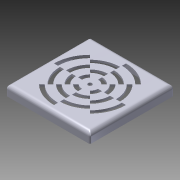
# Autodesk Inventor part: CompCellScopeArrayCover
Saved by Autodesk Inventor 2015 (Build 190159000, 159)
## iProperties
Created: 2015-03-24
Part Number: CompCellScopeArrayCover
Material: Generic
Document SubType Name: Modeling
Designer: Nitin
Density: 1 g/cm^3
Appearance: Default
Author: Nitin
Autodesk Inventor part; units mm, degrees
ref_plane "YZ Plane" through (0, 0, 0) normal (1, 0, 0) x (0, 1, 0)
ref_plane "XZ Plane" through (0, 0, 0) normal (0, 1, 0) x (-1, 0, 0)
ref_plane "XY Plane" through (0, 0, 0) normal (0, 0, 1) x (1, 0, 0)
sketch "Sketch1" plane through (0, 0, 0) normal (0, 1, 0) x (-1, 0, 0)
  line L0 (50, 50) -> (-50, 50)
  line L1 (-50, 50) -> (-50, -50)
  line L2 (-50, -50) -> (50, -50)
  line L3 (50, -50) -> (50, 50)
  line L4 (52.5, 52.5) -> (-52.5, 52.5)
  line L5 (-52.5, 52.5) -> (-52.5, -52.5)
  line L6 (-52.5, -52.5) -> (52.5, -52.5)
  line L7 (52.5, -52.5) -> (52.5, 52.5)
  point P0 (0, 0)
  dimension "d1" = 100
  dimension "d2" = 100
  dimension "d4" = 105
  dimension "d5" = 105
  constraints: 16 end point, 4 parallel, 2 horizontal, 2 perpendicular
  measures "d1" distance of L2.end L0.start
  measures "d2" distance of L1.end L2.end
  measures "d4" distance of L4.start L4.end
  measures "d5" distance of L4.end L5.end
extrude "Extrusion1" add sketch "Sketch1" against normal blind 10
extrude "Extrusion2" add sketch "Sketch1" along normal blind 2.5 contours L3 L2 L1 L0 | L7 L6 L5 L4
fillet "Fillet1" radius 2 1 edges at (52.5, -3.75, 52.5)
fillet "Fillet2" radius 2 1 edges at (-52.5, -3.75, 52.5)
fillet "Fillet3" radius 2 1 edges at (-52.5, -3.75, -52.5)
fillet "Fillet4" radius 2 1 edges at (52.5, -3.75, -52.5)
fillet "Fillet5" radius 5 8 edges at (0, 2.5, 52.5) (51.9142, 2.5, 51.9142) (52.5, 2.5, 0) (51.9142, 2.5, -51.9142) (0, 2.5, -52.5) (-51.9142, 2.5, -51.9142) (-52.5, 2.5, 0) (-51.9142, 2.5, 51.9142)
sketch "Sketch3" plane through (0, 2.5, 0) normal (0, 1, 0) x (1, 0, 0)
  circle A0 centre (0, 0) radius 45 construction
  circle A1 centre (0, 0) radius 40 construction
  circle A2 centre (0, 0) radius 37.5 construction
  circle A3 centre (0, 0) radius 32.5 construction
  circle A4 centre (0, 0) radius 30 construction
  circle A5 centre (0, 0) radius 25 construction
  circle A6 centre (0, 0) radius 22.5 construction
  circle A7 centre (0, 0) radius 17.5 construction
  line L0 (0, 0) -> (47.5, -47.5) construction
  line L1 (47.5, -47.5) -> (0, 0) construction
  line L2 (0, 0) -> (-50, 50) construction
  line L3 (0, 0) -> (-47.5, -47.5) construction
  line L4 (47.5, -47.5) -> (-47.5, -47.5) construction
  line L5 (0, 0) -> (47.5, 47.5) construction
  arc A8 (31.8198, -31.8198) -> (45, 0) centre (0, 0) ccw
  arc A9 (28.2843, -28.2843) -> (40, 0) centre (0, 0) ccw
  arc A10 (21.2132, -21.2132) -> (30, 0) centre (0, 0) ccw
  arc A11 (17.6777, -17.6777) -> (25, 0) centre (0, 0) ccw
  arc A12 (0, -32.5) -> (22.981, -22.981) centre (0, 0) ccw
  arc A13 (0, -37.5) -> (26.5165, -26.5165) centre (0, 0) ccw
  arc A14 (0, -17.5) -> (12.3744, -12.3744) centre (0, 0) ccw
  arc A15 (0, -22.5) -> (15.9099, -15.9099) centre (0, 0) ccw
  arc A16 (-21.2132, -21.2132) -> (0.0004, -30) centre (0, 0) ccw
  arc A17 (-17.6777, -17.6777) -> (0.0004, -25) centre (0, 0) ccw
  arc A18 (-31.8198, -31.8198) -> (0, -45) centre (0, 0) ccw
  arc A19 (-28.2843, -28.2843) -> (0, -40) centre (0, 0) ccw
  arc A20 (-37.5, 0) -> (-26.5165, -26.5165) centre (0, 0) ccw
  arc A21 (-32.5, 0) -> (-22.981, -22.981) centre (0, 0) ccw
  arc A22 (-17.5, 0) -> (-12.3744, -12.3744) centre (0, 0) ccw
  arc A23 (-22.5, 0) -> (-15.9099, -15.9099) centre (0, 0) ccw
  arc A24 (37.5, 0) -> (26.5165, 26.5165) centre (0, 0) ccw
  arc A25 (32.5, 0) -> (22.981, 22.981) centre (0, 0) ccw
  arc A26 (22.5, 0) -> (15.9099, 15.9099) centre (0, 0) ccw
  arc A27 (17.5, 0) -> (12.3744, 12.3744) centre (0, 0) ccw
  arc A28 (28.2843, 28.2843) -> (0, 40) centre (0, 0) ccw
  arc A29 (31.8198, 31.8198) -> (0, 45) centre (0, 0) ccw
  arc A30 (17.6777, 17.6777) -> (0, 25) centre (0, 0) ccw
  arc A31 (21.2132, 21.2132) -> (0, 30) centre (0, 0) ccw
  arc A32 (0, 32.5) -> (-22.981, 22.981) centre (0, 0) ccw
  arc A33 (0, 37.5) -> (-26.5165, 26.5165) centre (0, 0) ccw
  arc A34 (0, 17.5) -> (-12.3744, 12.3744) centre (0, 0) ccw
  arc A35 (0, 22.5) -> (-15.9099, 15.9099) centre (0, 0) ccw
  arc A36 (-17.6777, 17.6777) -> (-25, 0) centre (0, 0) ccw
  arc A37 (-21.2132, 21.2132) -> (-30, 0) centre (0, 0) ccw
  arc A38 (-28.2843, 28.2843) -> (-40, 0) centre (0, 0) ccw
  arc A39 (-31.8198, 31.8198) -> (-45, 0) centre (0, 0) ccw
  line L6 (45, 0) -> (40, 0)
  line L7 (47.5, 47.5) -> (47.5, -47.5) projected
  line L8 (37.5, 0) -> (32.5, 0)
  line L9 (30, 0) -> (25, 0)
  line L10 (22.5, 0) -> (17.5, 0)
  line L11 (31.8198, -31.8198) -> (28.2843, -28.2843)
  line L12 (26.5165, -26.5165) -> (22.981, -22.981)
  line L13 (21.2132, -21.2132) -> (17.6777, -17.6777)
  line L14 (15.9099, -15.9099) -> (12.3744, -12.3744)
  line L15 (0, -45) -> (0, -40)
  line L16 (0, -37.5) -> (0, -32.5)
  line L17 (0.0004, -30) -> (0.0004, -25)
  line L18 (0, -22.5) -> (0, -17.5)
  line L19 (-31.8198, -31.8198) -> (-28.2843, -28.2843)
  line L20 (-26.5165, -26.5165) -> (-22.981, -22.981)
  line L21 (-21.2132, -21.2132) -> (-17.6777, -17.6777)
  line L22 (-15.9099, -15.9099) -> (-12.3744, -12.3744)
  line L23 (-45, 0) -> (-40, 0)
  line L24 (-37.5, 0) -> (-32.5, 0)
  line L25 (-30, 0) -> (-25, 0)
  line L26 (-22.5, 0) -> (-17.5, 0)
  line L27 (-31.8198, 31.8198) -> (-28.2843, 28.2843)
  line L28 (-26.5165, 26.5165) -> (-22.981, 22.981)
  line L29 (-21.2132, 21.2132) -> (-17.6777, 17.6777)
  line L30 (-15.9099, 15.9099) -> (-12.3744, 12.3744)
  line L31 (0, 45) -> (0, 40)
  line L32 (0, 37.5) -> (0, 32.5)
  line L33 (0, 30) -> (0, 25)
  line L34 (0, 22.5) -> (0, 17.5)
  line L35 (31.8198, 31.8198) -> (28.2843, 28.2843)
  line L36 (26.5165, 26.5165) -> (22.981, 22.981)
  line L37 (21.2132, 21.2132) -> (17.6777, 17.6777)
  line L38 (15.9099, 15.9099) -> (12.3744, 12.3744)
  circle A40 centre (0, 0) radius 15 construction
  circle A41 centre (0, 0) radius 10 construction
  circle A42 centre (0, 0) radius 7.5 construction
  circle A43 centre (0, 0) radius 2.5 construction
  arc A44 (-10.6066, -10.6066) -> (0, -15) centre (0, 0) ccw
  arc A45 (-7.0711, -7.0711) -> (0, -10) centre (0, 0) ccw
  arc A46 (7.0711, 7.0711) -> (0.075, 9.9997) centre (0, 0) ccw
  arc A47 (10.6066, 10.6066) -> (0.075, 14.9998) centre (0, 0) ccw
  arc A48 (-7.0711, 7.0711) -> (-10, 0) centre (0, 0) ccw
  arc A49 (-10.6066, 10.6066) -> (-15, 0) centre (0, 0) ccw
  arc A50 (7.0711, -7.0711) -> (10, 0) centre (0, 0) ccw
  arc A51 (10.6066, -10.6066) -> (15, 0) centre (0, 0) ccw
  line L39 (-10.6066, -10.6066) -> (-7.0711, -7.0711)
  line L40 (0, -15) -> (0, -10)
  line L41 (10.6066, -10.6066) -> (7.0711, -7.0711)
  line L42 (10, 0) -> (15, 0)
  line L43 (7.0711, 7.0711) -> (10.6066, 10.6066)
  line L44 (0.075, 9.9997) -> (0.075, 14.9998)
  line L45 (-7.0711, 7.0711) -> (-10.6066, 10.6066)
  line L46 (-10, 0) -> (-15, 0)
  circle A52 centre (0, 0) radius 2.5
  dimension "d23" = 90
  dimension "d24" = 80
  dimension "d25" = 75
  dimension "d26" = 65
  dimension "d27" = 60
  dimension "d28" = 50
  dimension "d29" = 45
  dimension "d30" = 35
  dimension "d31" = 30
  dimension "d32" = 20
  dimension "d33" = 15
  dimension "d34" = 5
  constraints: 84 point on circle, 83 end point, 43 centre point, 15 collinear, 13 coincident, 8 perpendicular, 2 parallel, 1 concentric, 1 vertical, 210 other
  measures "d33" diameter of A42
  measures "d34" diameter of A43
extrude "Extrusion3" cut sketch "Sketch3" against normal blind 2.5
body "Solid1"
